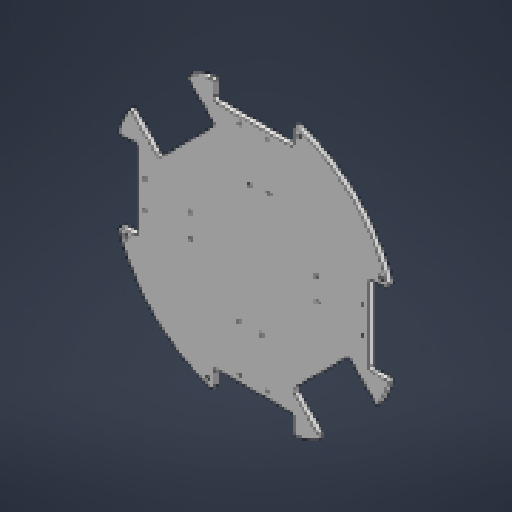
# Autodesk Inventor part: SecondPlate
Saved by Autodesk Inventor 2024.2 (Build 282272000, 272)
## iProperties
Created: 2023-12-22
Part Number: SecondPlate
Material: 一般
Document SubType Name: Modeling
Designer: Hanaoka
Density: 1 g/cm^3
Appearance: 既定
Author: Hanaoka
Autodesk Inventor part; units mm, degrees
ref_plane "YZ Plane" through (0, 0, 0) normal (1, 0, 0) x (0, 1, 0)
ref_plane "XZ Plane" through (0, 0, 0) normal (0, 1, 0) x (-1, 0, 0)
ref_plane "XY Plane" through (0, 0, 0) normal (0, 0, 1) x (1, 0, 0)
sketch "スケッチ1" plane through (0, 0, 0) normal (0, 0, 1) x (1, 0, 0)
  arc A0 (4.2199, -1.5405) -> (-52.5892, 55.2686) centre (-79.5487, -28.5) ccw projected
  arc A1 (2.792, -3.5) -> (4.2199, -1.5405) centre (2.792, -2) ccw projected
  line L0 (-5.5487, -3.5) -> (2.792, -3.5) projected
  circle A2 centre (0, 0) radius 2.5 projected
  circle A3 centre (0, 0) radius 1.3 projected
  arc A4 (-5.5487, -3.5) -> (-7.5487, -5.5) centre (-5.5487, -5.5) ccw projected
  line L1 (-7.5487, -51.5) -> (-7.5487, -5.5) projected
  arc A5 (-7.5487, -51.5) -> (-5.5487, -53.5) centre (-5.5487, -51.5) ccw projected
  line L2 (2.792, -53.5) -> (-5.5487, -53.5) projected
  arc A6 (4.2199, -55.4595) -> (2.792, -53.5) centre (2.792, -55) ccw projected
  arc A7 (-1.2521, -68.6701) -> (4.2199, -55.4595) centre (-79.5487, -28.5) ccw projected
  arc A8 (-3.6474, -69.046) -> (-1.2521, -68.6701) centre (-2.5867, -67.9854) ccw projected
  line L3 (-9.6341, -63.0593) -> (-3.6474, -69.046) projected
  arc A9 (-9.6341, -63.0593) -> (-13.8768, -63.0593) centre (-11.7555, -65.1806) ccw projected
  line L4 (-15.9981, -65.1806) -> (-13.8768, -63.0593) projected
  line L5 (-39.3326, -88.5151) -> (-19.5336, -68.7161) projected
  line L6 (-44.9895, -94.172) -> (-42.8682, -92.0506) projected
  arc A10 (-44.9895, -94.172) -> (-44.9895, -98.4146) centre (-42.8682, -96.2933) ccw projected
  line L7 (-39.0027, -104.4014) -> (-44.9895, -98.4146) projected
  arc A11 (-39.3786, -106.7966) -> (-39.0027, -104.4014) centre (-40.0634, -105.462) ccw projected
  arc A12 (-52.5892, -112.2686) -> (-39.3786, -106.7966) centre (-79.5487, -28.5) ccw projected
  arc A13 (-54.5487, -110.8408) -> (-52.5892, -112.2686) centre (-53.0487, -110.8408) ccw projected
  line L8 (-54.5487, -102.5) -> (-54.5487, -110.8408) projected
  arc A14 (-54.5487, -102.5) -> (-56.5487, -100.5) centre (-56.5487, -102.5) ccw projected
  line L9 (-102.5487, -100.5) -> (-56.5487, -100.5) projected
  arc A15 (-102.5487, -100.5) -> (-104.5487, -102.5) centre (-102.5487, -102.5) ccw projected
  line L10 (-104.5487, -110.8408) -> (-104.5487, -102.5) projected
  arc A16 (-106.5083, -112.2686) -> (-104.5487, -110.8408) centre (-106.0487, -110.8408) ccw projected
  arc A17 (-163.3174, -55.4595) -> (-106.5083, -112.2686) centre (-79.5487, -28.5) ccw projected
  circle A18 centre (-108.0487, -108.0487) radius 2.5 projected
  circle A19 centre (-108.0487, -108.0487) radius 1.3 projected
  arc A20 (-161.8895, -53.5) -> (-163.3174, -55.4595) centre (-161.8895, -55) ccw projected
  line L11 (-153.5487, -53.5) -> (-161.8895, -53.5) projected
  circle A21 centre (-159.0975, -57) radius 1.3 projected
  circle A22 centre (-159.0975, -57) radius 2.5 projected
  arc A23 (-153.5487, -53.5) -> (-151.5487, -51.5) centre (-153.5487, -51.5) ccw projected
  line L12 (-151.5487, -5.5) -> (-151.5487, -51.5) projected
  line L13 (-161.8895, -3.5) -> (-153.5487, -3.5) projected
  arc A24 (-151.5487, -5.5) -> (-153.5487, -3.5) centre (-153.5487, -5.5) ccw projected
  arc A25 (-163.3174, -1.5405) -> (-161.8895, -3.5) centre (-161.8895, -2) ccw projected
  arc A26 (-157.8454, 11.6701) -> (-163.3174, -1.5405) centre (-79.5487, -28.5) ccw projected
  arc A27 (-155.4501, 12.046) -> (-157.8454, 11.6701) centre (-156.5108, 10.9854) ccw projected
  line L14 (-149.4633, 6.0593) -> (-155.4501, 12.046) projected
  arc A28 (-149.4633, 6.0593) -> (-145.2207, 6.0593) centre (-147.342, 8.1806) ccw projected
  line L15 (-143.0994, 8.1806) -> (-145.2207, 6.0593) projected
  line L16 (-119.7648, 31.5151) -> (-139.5638, 11.7161) projected
  line L17 (-114.108, 37.172) -> (-116.2293, 35.0506) projected
  arc A29 (-114.108, 37.172) -> (-114.108, 41.4146) centre (-116.2293, 39.2933) ccw projected
  line L18 (-120.0948, 47.4014) -> (-114.108, 41.4146) projected
  arc A30 (-119.7188, 49.7966) -> (-120.0948, 47.4014) centre (-119.0341, 48.462) ccw projected
  arc A31 (-106.5083, 55.2686) -> (-119.7188, 49.7966) centre (-79.5487, -28.5) ccw projected
  arc A32 (-104.5487, 53.8408) -> (-106.5083, 55.2686) centre (-106.0487, 53.8408) ccw projected
  line L19 (-104.5487, 45.5) -> (-104.5487, 53.8408) projected
  arc A33 (-104.5487, 45.5) -> (-102.5487, 43.5) centre (-102.5487, 45.5) ccw projected
  line L20 (-56.5487, 43.5) -> (-102.5487, 43.5) projected
  arc A34 (-52.5892, 55.2686) -> (-54.5487, 53.8408) centre (-53.0487, 53.8408) ccw projected
  line L21 (-54.5487, 53.8408) -> (-54.5487, 45.5) projected
  arc A35 (-56.5487, 43.5) -> (-54.5487, 45.5) centre (-56.5487, 45.5) ccw projected
  circle A36 centre (-51.0487, 51.0487) radius 2.5 projected
  circle A37 centre (-51.0487, 51.0487) radius 1.3 projected
  circle A38 centre (-11.5487, -37) radius 0.8 projected
  circle A39 centre (-11.5487, -20) radius 0.8 projected
  line L22 (-9.5487, -39.5) -> (-9.5487, -17.5) projected
  line L23 (-9.5487, -17.5) -> (-13.5487, -17.5) projected
  line L24 (-13.5487, -39.5) -> (-13.5487, -17.5) projected
  line L25 (-9.5487, -39.5) -> (-13.5487, -39.5) projected
  circle A40 centre (-71.0487, 39.5) radius 0.8 projected
  circle A41 centre (-88.0487, 39.5) radius 0.8 projected
  line L26 (-68.5487, 41.5) -> (-90.5487, 41.5) projected
  line L27 (-90.5487, 41.5) -> (-90.5487, 37.5) projected
  line L28 (-68.5487, 37.5) -> (-90.5487, 37.5) projected
  line L29 (-68.5487, 41.5) -> (-68.5487, 37.5) projected
  circle A42 centre (-147.5487, -20) radius 0.8 projected
  circle A43 centre (-147.5487, -37) radius 0.8 projected
  line L30 (-149.5487, -17.5) -> (-149.5487, -39.5) projected
  line L31 (-149.5487, -39.5) -> (-145.5487, -39.5) projected
  line L32 (-145.5487, -17.5) -> (-145.5487, -39.5) projected
  line L33 (-149.5487, -17.5) -> (-145.5487, -17.5) projected
  circle A44 centre (-88.0487, -96.5) radius 0.8 projected
  circle A45 centre (-71.0487, -96.5) radius 0.8 projected
  line L34 (-90.5487, -98.5) -> (-68.5487, -98.5) projected
  line L35 (-68.5487, -98.5) -> (-68.5487, -94.5) projected
  line L36 (-90.5487, -94.5) -> (-68.5487, -94.5) projected
  line L37 (-90.5487, -98.5) -> (-90.5487, -94.5) projected
  line L38 (-116.2293, 35.0506) -> (-119.7648, 31.5151)
  line L39 (-139.5638, 11.7161) -> (-143.0994, 8.1806)
  line L40 (-15.9981, -65.1806) -> (-19.5336, -68.7161)
  line L41 (-42.8682, -92.0506) -> (-42.6896, -91.8721)
  line L42 (-42.6896, -91.8721) -> (-39.3326, -88.5151)
  line L43 (-49.5487, 45.911) -> (-49.5487, 38)
  line L44 (-51.5487, 36) -> (-86.1672, 36)
  line L45 (-87.5815, 35.4142) -> (-143.4629, -20.4673)
  line L46 (-5.1377, 1.5) -> (-13.0487, 1.5)
  line L47 (-15.0487, -0.5) -> (-15.0487, -35.1185)
  line L48 (-15.6345, -36.5327) -> (-71.516, -92.4142)
  arc A46 (-3.3004, 4.2901) -> (-46.7586, 47.7483) centre (-79.5487, -28.5) ccw
  arc A47 (-5.1377, 1.5) -> (-3.3004, 4.2901) centre (-5.1377, 3.5) ccw
  arc A48 (-46.7586, 47.7483) -> (-49.5487, 45.911) centre (-47.5487, 45.911) ccw
  arc A49 (-51.5487, 36) -> (-49.5487, 38) centre (-51.5487, 38) ccw
  arc A50 (-13.0487, 1.5) -> (-15.0487, -0.5) centre (-13.0487, -0.5) ccw
  arc A51 (-15.6345, -36.5327) -> (-15.0487, -35.1185) centre (-17.0487, -35.1185) ccw
  arc A52 (-86.1672, 36) -> (-87.5815, 35.4142) centre (-86.1672, 34) ccw
  line L49 (-129.6643, 21.6156) -> (-29.4331, -78.6156) construction
  line L50 (-153.9597, -58.5) -> (-146.0487, -58.5)
  line L51 (-144.0487, -56.5) -> (-144.0487, -21.8815)
  line L52 (-109.5487, -102.911) -> (-109.5487, -95)
  line L53 (-107.5487, -93) -> (-72.9302, -93)
  arc A53 (-155.7971, -61.2901) -> (-112.3389, -104.7483) centre (-79.5487, -28.5) ccw
  arc A54 (-112.3389, -104.7483) -> (-109.5487, -102.911) centre (-111.5487, -102.911) ccw
  arc A55 (-153.9597, -58.5) -> (-155.7971, -61.2901) centre (-153.9597, -60.5) ccw
  arc A56 (-146.0487, -58.5) -> (-144.0487, -56.5) centre (-146.0487, -56.5) ccw
  arc A57 (-107.5487, -93) -> (-109.5487, -95) centre (-107.5487, -95) ccw
  arc A58 (-72.9302, -93) -> (-71.516, -92.4142) centre (-72.9302, -91) ccw
  arc A59 (-143.4629, -20.4673) -> (-144.0487, -21.8815) centre (-142.0487, -21.8815) ccw
  line L54 (-9.6341, -63.0593) -> (-18.8265, -53.8669)
  line L55 (-21.6549, -53.8669) -> (-54.1819, -86.3938)
  line L56 (-54.1819, -89.2222) -> (-44.9895, -98.4146)
  arc A60 (-18.8265, -53.8669) -> (-21.6549, -53.8669) centre (-20.2407, -55.2811) ccw
  arc A61 (-54.1819, -86.3938) -> (-54.1819, -89.2222) centre (-52.7676, -87.808) ccw
  line L57 (-114.108, 41.4146) -> (-104.9156, 32.2222)
  line L58 (-104.9156, 29.3938) -> (-137.4425, -3.1331)
  line L59 (-140.2709, -3.1331) -> (-149.4633, 6.0593)
  arc A62 (-104.9156, 29.3938) -> (-104.9156, 32.2222) centre (-106.3298, 30.808) ccw
  arc A63 (-140.2709, -3.1331) -> (-137.4425, -3.1331) centre (-138.8567, -1.7189) ccw
  point P0 (0, 0)
  point P1 (-49.5487, 48.8886)
  point P2 (-2.1601, 1.5)
  point P3 (-2.1601, 1.5)
  point P4 (-49.5487, 48.8886)
  point P5 (-55.5961, -87.808)
  dimension "d2" = 5
  dimension "d3" = 2
  dimension "d4" = 5
  dimension "d5" = 5
  dimension "d6" = 1.5
  dimension "d7" = 1.5
  dimension "d8" = 20
  dimension "d9" = 20
  dimension "d12" = 15
  dimension "d13" = 2
  constraints: 44 end point, 40 point on circle, 20 tangent, 18 centre point, 18 symmetric about line, 11 parallel, 8 equal radius, 7 point on line, 4 collinear, 2 midpoint, 1 coincident, 1 perpendicular, 7 other
  measures "d2" radial gap between concentric circles of A0 A46
  measures "d3" radius of A47
  measures "d4" distance between parallel lines of L0 L46
  measures "d5" distance between parallel lines of L21 L43
  measures "d6" distance between parallel lines of L44 L28
  measures "d7" distance between parallel lines of L47 L24
  measures "d8" distance between parallel lines of L16 L45
  measures "d9" distance between parallel lines of L5 L48
  measures "d12" distance of point (-55.596, -87.808) L7.end
  measures "d13" radius of A60
extrude "押し出し1" add sketch "スケッチ1" along normal blind 1 contours A1 L0 A4 L1 A5 L2 A6 A7 A8 L3 L54 A60 L55 A61 L56 L7 A11 A12 A13 L8 A14 L9 A15 L10 A16 A17 A20 L11 A23 L12 A24 L13 A25 A26 A27 L14 L59 A63 L58 A62 L57 L18 A30 A31 A32 L19 A33 L20 A35 L21 A34 A0 | A2 | A18 | A22 | A36 | L25 L24 L23 L22 | L29 L28 L27 L26 | L33 L32 L31 L30 | L37 L36 L35 L34 | A48 A46 A47 L46 A50 L47 A51 L48 A58 L53 A57 L52 A54 A53 A55 L50 A56 L51 A59 L45 A52 L44 A49 L43
sketch "スケッチ2" plane through (0, 0, 0) normal (0, 0, -1) x (-1, 0, 0)
  arc A0 (-4.2199, -1.5405) -> (-2.792, -3.5) centre (-2.792, -2) ccw projected
  line L0 (5.5487, -3.5) -> (-2.792, -3.5) projected
  arc A1 (7.5487, -5.5) -> (5.5487, -3.5) centre (5.5487, -5.5) ccw projected
  line L1 (7.5487, -51.5) -> (7.5487, -5.5) projected
  arc A2 (5.5487, -53.5) -> (7.5487, -51.5) centre (5.5487, -51.5) ccw projected
  line L2 (-2.792, -53.5) -> (5.5487, -53.5) projected
  arc A3 (-2.792, -53.5) -> (-4.2199, -55.4595) centre (-2.792, -55) ccw projected
  arc A4 (-4.2199, -55.4595) -> (1.2521, -68.6701) centre (79.5487, -28.5) ccw projected
  arc A5 (1.2521, -68.6701) -> (3.6474, -69.046) centre (2.5867, -67.9854) ccw projected
  line L3 (18.8265, -53.8669) -> (3.6474, -69.046) projected
  line L4 (39.0027, -104.4014) -> (54.1819, -89.2222) projected
  arc A6 (39.0027, -104.4014) -> (39.3786, -106.7966) centre (40.0634, -105.462) ccw projected
  arc A7 (39.3786, -106.7966) -> (52.5892, -112.2686) centre (79.5487, -28.5) ccw projected
  arc A8 (52.5892, -112.2686) -> (54.5487, -110.8408) centre (53.0487, -110.8408) ccw projected
  line L5 (54.5487, -102.5) -> (54.5487, -110.8408) projected
  arc A9 (56.5487, -100.5) -> (54.5487, -102.5) centre (56.5487, -102.5) ccw projected
  line L6 (102.5487, -100.5) -> (56.5487, -100.5) projected
  arc A10 (104.5487, -102.5) -> (102.5487, -100.5) centre (102.5487, -102.5) ccw projected
  line L7 (104.5487, -110.8408) -> (104.5487, -102.5) projected
  arc A11 (104.5487, -110.8408) -> (106.5083, -112.2686) centre (106.0487, -110.8408) ccw projected
  arc A12 (106.5083, -112.2686) -> (163.3174, -55.4595) centre (79.5487, -28.5) ccw projected
  arc A13 (163.3174, -55.4595) -> (161.8895, -53.5) centre (161.8895, -55) ccw projected
  line L8 (153.5487, -53.5) -> (161.8895, -53.5) projected
  arc A14 (151.5487, -51.5) -> (153.5487, -53.5) centre (153.5487, -51.5) ccw projected
  line L9 (151.5487, -5.5) -> (151.5487, -51.5) projected
  arc A15 (153.5487, -3.5) -> (151.5487, -5.5) centre (153.5487, -5.5) ccw projected
  line L10 (161.8895, -3.5) -> (153.5487, -3.5) projected
  arc A16 (161.8895, -3.5) -> (163.3174, -1.5405) centre (161.8895, -2) ccw projected
  arc A17 (163.3174, -1.5405) -> (157.8454, 11.6701) centre (79.5487, -28.5) ccw projected
  arc A18 (157.8454, 11.6701) -> (155.4501, 12.046) centre (156.5108, 10.9854) ccw projected
  line L11 (140.2709, -3.1331) -> (155.4501, 12.046) projected
  line L12 (120.0948, 47.4014) -> (104.9156, 32.2222) projected
  arc A19 (120.0948, 47.4014) -> (119.7188, 49.7966) centre (119.0341, 48.462) ccw projected
  arc A20 (119.7188, 49.7966) -> (106.5083, 55.2686) centre (79.5487, -28.5) ccw projected
  arc A21 (106.5083, 55.2686) -> (104.5487, 53.8408) centre (106.0487, 53.8408) ccw projected
  line L13 (104.5487, 45.5) -> (104.5487, 53.8408) projected
  arc A22 (102.5487, 43.5) -> (104.5487, 45.5) centre (102.5487, 45.5) ccw projected
  line L14 (56.5487, 43.5) -> (102.5487, 43.5) projected
  arc A23 (54.5487, 45.5) -> (56.5487, 43.5) centre (56.5487, 45.5) ccw projected
  line L15 (54.5487, 53.8408) -> (54.5487, 45.5) projected
  arc A24 (54.5487, 53.8408) -> (52.5892, 55.2686) centre (53.0487, 53.8408) ccw projected
  arc A25 (52.5892, 55.2686) -> (-4.2199, -1.5405) centre (79.5487, -28.5) ccw projected
  circle A26 centre (0, 0) radius 1.3 projected
  circle A27 centre (108.0487, -108.0487) radius 1.3 projected
  circle A28 centre (159.0975, -57) radius 1.3 projected
  circle A29 centre (51.0487, 51.0487) radius 1.3 projected
  circle A30 centre (11.5487, -37) radius 0.8 projected
  circle A31 centre (11.5487, -20) radius 0.8 projected
  circle A32 centre (71.0487, 39.5) radius 0.8 projected
  circle A33 centre (88.0487, 39.5) radius 0.8 projected
  circle A34 centre (147.5487, -20) radius 0.8 projected
  circle A35 centre (147.5487, -37) radius 0.8 projected
  circle A36 centre (71.0487, -96.5) radius 0.8 projected
  circle A37 centre (88.0487, -96.5) radius 0.8 projected
  line L16 (68.5487, 37.5) -> (90.5487, 37.5) projected
  line L17 (68.5487, 41.5) -> (90.5487, 41.5) projected
  line L18 (90.5487, 41.5) -> (90.5487, 37.5) projected
  line L19 (68.5487, 41.5) -> (68.5487, 37.5) projected
  line L20 (149.5487, -17.5) -> (149.5487, -39.5) projected
  line L21 (149.5487, -17.5) -> (145.5487, -17.5) projected
  line L22 (145.5487, -17.5) -> (145.5487, -39.5) projected
  line L23 (149.5487, -39.5) -> (145.5487, -39.5) projected
  line L24 (90.5487, -98.5) -> (68.5487, -98.5) projected
  line L25 (90.5487, -94.5) -> (68.5487, -94.5) projected
  line L26 (90.5487, -98.5) -> (90.5487, -94.5) projected
  line L27 (68.5487, -98.5) -> (68.5487, -94.5) projected
  line L28 (13.5487, -39.5) -> (13.5487, -17.5) projected
  line L29 (9.5487, -17.5) -> (13.5487, -17.5) projected
  line L30 (9.5487, -39.5) -> (9.5487, -17.5) projected
  line L31 (9.5487, -39.5) -> (13.5487, -39.5) projected
  arc A38 (21.6549, -53.8669) -> (18.8265, -53.8669) centre (20.2407, -55.2811) ccw projected
  line L32 (54.1819, -86.3938) -> (21.6549, -53.8669) projected
  arc A39 (54.1819, -89.2222) -> (54.1819, -86.3938) centre (52.7676, -87.808) ccw projected
  arc A40 (137.4425, -3.1331) -> (140.2709, -3.1331) centre (138.8567, -1.7189) ccw projected
  line L33 (104.9156, 29.3938) -> (137.4425, -3.1331) projected
  arc A41 (104.9156, 32.2222) -> (104.9156, 29.3938) centre (106.3298, 30.808) ccw projected
  circle A42 centre (51.0487, 51.0487) radius 2.5
  circle A43 centre (0, 0) radius 2.5
  circle A44 centre (159.0975, -57) radius 2.5
  circle A45 centre (108.0487, -108.0487) radius 2.5
  line L34 (17.3233, 33.7254) -> (141.7741, -90.7254) construction
  circle A46 centre (118.7932, -38.0459) radius 1.1
  circle A47 centre (89.0947, -67.7444) radius 1.1
  line L35 (118.7932, -38.0459) -> (89.0947, -67.7444) construction
  line L36 (121.179, 13.1303) -> (37.9184, -70.1303) construction
  circle A48 centre (70.0028, 10.7444) radius 1.1
  circle A49 centre (40.3043, -18.9541) radius 1.1
  line L37 (70.0028, 10.7444) -> (40.3043, -18.9541) construction
  point P0 (0, 0)
  point P1 (103.9439, -52.8952)
  point P2 (79.5487, -28.5)
  dimension "d16" = 5
  dimension "d17" = 2.2
  dimension "d18" = 42
  dimension "d19" = 34.5
  dimension "d20" = 34.5
  constraints: 8 centre point, 8 end point, 5 equal radius, 4 coincident, 4 midpoint, 2 point on circle, 1 parallel, 2 other
  measures "d16" diameter of A42
  measures "d17" diameter of A47
  measures "d18" distance of L35.start L35.end
  measures "d19" distance of point (103.944, -52.895) point (79.549, -28.5)
  measures "d20" distance between parallel lines of L36 L37
extrude "押し出し2" add sketch "スケッチ2" along normal blind 2 contours A25 A24 L15 A23 L14 A22 L13 A21 A20 A19 L12 A41 L33 A40 L11 A18 A17 A16 L10 A15 L9 A14 L8 A13 A12 A11 L7 A10 L6 A9 L5 A8 A7 A6 L4 A39 L32 A38 L3 A5 A4 A3 L2 A2 L1 A1 L0 A0 | A46 | A47 | A48 | A49
extrude "押し出し3" cut sketch "スケッチ2" along normal mid plane 5 contours A46 | A47 | A48 | A49
sketch "スケッチ3" plane through (0, 0, 1) normal (0, 0, 1) x (1, 0, 0)
  circle A0 centre (-39.861, -32.8324) radius 1.1
  circle A1 centre (-75.2164, -68.1877) radius 1.1
  circle A2 centre (-82.2874, 9.594) radius 1.1
  circle A3 centre (-119.2364, -24.1676) radius 1.1
  line L0 (-82.2874, 9.594) -> (-39.861, -32.8324) construction
  line L1 (-39.861, -32.8324) -> (-75.2164, -68.1877) construction
  line L2 (-75.2164, -68.1877) -> (-119.2364, -24.1676) construction
  line L3 (-119.2364, -24.1676) -> (-83.8811, 11.1877) construction
  line L4 (-17.3233, 33.7254) -> (-141.7741, -90.7254) construction
  arc A4 (4.2199, -1.5405) -> (-52.5892, 55.2686) centre (-79.5487, -28.5) ccw projected
  arc A5 (-163.3174, -55.4595) -> (-106.5083, -112.2686) centre (-79.5487, -28.5) ccw projected
  line L5 (-104.9156, 29.3938) -> (-137.4425, -3.1331) projected
  line L6 (-121.179, 13.1303) -> (-37.9184, -70.1303) construction
  line L7 (-54.1819, -86.3938) -> (-21.6549, -53.8669) projected
  circle A6 centre (-39.861, -32.8324) radius 2.5
  circle A7 centre (-75.2164, -68.1877) radius 2.5
  circle A8 centre (-119.2364, -24.1676) radius 2.5
  circle A9 centre (-82.2874, 9.594) radius 2.5
  point P0 (0, 0)
  point P1 (-57.5387, -50.51)
  point P2 (-97.2264, -46.1777)
  dimension "d23" = 2.2
  dimension "d24" = 50
  dimension "d25" = 60
  dimension "d26" = 5
  constraints: 12 end point, 8 centre point, 6 equal radius, 4 coincident, 4 midpoint, 4 parallel, 3 point on line, 2 point on circle
  measures "d23" diameter of A1
  measures "d24" distance of L0.end L1.end
  measures "d25" distance of L0.start L0.end
  measures "d26" diameter of A7
extrude "押し出し4" cut sketch "スケッチ3" against normal up to surface (3 mm away) contours A0 | A1 | A2 | A3
equation "\"d5\" = d4"
equation "\"d7\" = d6"
equation "\"d8\" = d9"
equation "\"d20\" = d19"
